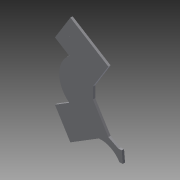
# Autodesk Inventor part: drzak_buzirka
Saved by Autodesk Inventor 2015 (Build 190159000, 159)
## iProperties
Created: 2016-01-15
Part Number: drzak_buzirka
Material: Generic
Document SubType Name: Modeling
Designer: Turboslimak
Density: 1 g/cm^3
Appearance: Default
Author: Turboslimak
Autodesk Inventor part; units mm, degrees
ref_plane "YZ Plane" through (0, 0, 0) normal (1, 0, 0) x (0, 1, 0)
ref_plane "XZ Plane" through (0, 0, 0) normal (0, 1, 0) x (-1, 0, 0)
ref_plane "XY Plane" through (0, 0, 0) normal (0, 0, 1) x (1, 0, 0)
sketch "Sketch1" plane through (0, 0, 0) normal (0, 1, 0) x (-1, 0, 0)
  line L0 (-21, -5) -> (-21, 5)
  line L1 (0, -18) -> (-21, -5)
  line L2 (0, 18) -> (-21, 5)
  line L3 (-21, -5) -> (-34.6852, -27.1069)
  line L4 (0, -18) -> (-13.6852, -40.1069)
  line L5 (-13.6852, -40.1069) -> (-34.6852, -27.1069)
  line L6 (-21, 5) -> (-34.6852, 27.1069)
  line L7 (0, 18) -> (-13.6852, 40.1069)
  line L8 (-13.6852, 40.1069) -> (-34.6852, 27.1069)
  arc A0 (0, -18) -> (0, 18) centre (-13.5, 0) ccw
  circle A1 centre (0, 0) radius 0.1
  line L9 (-13.6852, -40.1069) -> (0, -18)
  line L10 (0, -18) -> (12.754, -25.8953)
  line L11 (12.754, -25.8953) -> (-0.9312, -48.0022)
  line L12 (-0.9312, -48.0022) -> (-13.6852, -40.1069)
  line L13 (0, 18) -> (-13.6852, 40.1069)
  line L14 (-13.6852, 40.1069) -> (-0.9312, 48.0022)
  line L15 (-0.9312, 48.0022) -> (12.754, 25.8953)
  line L16 (12.754, 25.8953) -> (0, 18)
  line L17 (-34.6852, -27.1069) -> (-43.636, -31.5659)
  line L18 (-44.556, -41.5235) -> (-43.636, -31.5659)
  arc A2 (-26.1826, -32.3704) -> (-44.556, -41.5235) centre (-28.2096, -51.3191) ccw
  line L19 (-26.1826, -32.3704) -> (-34.6852, -27.1069)
  line L20 (-34.6852, -27.1069) -> (-43.636, -31.5659)
  line L21 (-43.636, -31.5659) -> (-44.556, -41.5235)
  arc A3 (-26.1826, -32.3704) -> (-44.556, -41.5235) centre (-28.2096, -51.3191) ccw
  line L22 (-43.636, -31.5659) -> (-46.6233, -31.2899)
  line L23 (-44.556, -41.5235) -> (-47.5433, -41.2475)
  line L24 (-47.5433, -41.2475) -> (-46.6233, -31.2899)
  line L25 (5.9114, -36.9488) -> (-6.8426, -29.0534)
  line L26 (5.9114, 36.9488) -> (-6.8426, 29.0534)
  circle A4 centre (-0.4656, -33.0011) radius 0.1
  circle A5 centre (-0.4656, 33.0011) radius 0.1
  point P0 (-21, 0)
  point P1 (-39.1606, -29.3364)
  dimension "d5" = 10
  dimension "d6" = 26
  dimension "d7" = 26
  dimension "d8" = 26
  dimension "d9" = 26
  dimension "d10" = 36
  dimension "d12" = 0.2
  dimension "d13" = 15
  dimension "d14" = 15
  dimension "d22" = 3
  dimension "d25" = 0.2
  dimension "d26" = 0.2
  constraints: 54 end point, 8 perpendicular, 7 midpoint, 6 centre point, 6 point on circle, 5 collinear, 4 parallel, 1 point on line, 1 other
  measures "d5" distance of L0.start L0.end
  measures "d6" distance of L0.start L3.end
  measures "d7" distance of L1.start L4.end
  measures "d8" distance of L2.start L7.end
  measures "d9" distance of L0.end L6.end
  measures "d10" distance of L1.start L2.start
  measures "d12" diameter of A1
  measures "d13" distance of L1.start L10.end
  measures "d14" distance of L7.end L14.end
  measures "d22" distance of L17.end L22.end
  measures "d25" diameter of A4
  measures "d26" diameter of A5
extrude "Extrusion1" add sketch "Sketch1" along normal blind 2 contours L0 L2 A0 L1 | L1 L4 L5 L3 | L6 L8 L7 L2 | L10 L11 L25 A4 L4 | L7 L26 A5 L15 L16 | L25 A4 L11 L12 L4 | L7 L14 L15 L26 A5 | A4 L25 | L25 A4 | A5 L26 | L26 A5
extrude "Extrusion2" add sketch "Sketch1" along normal blind 2 contours L5 A2 L18 L17
extrude "Extrusion3" add sketch "Sketch1" along normal blind 2 contours L18 L23 L24 L22
extrude "Extrusion4" cut sketch "Sketch1" along normal blind 2 contours A4 L25 | L25 A4 | A5 L26 | L26 A5
body "Solid1"
